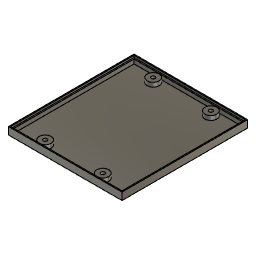
VersaTermBottom (Autodesk Fusion 360 design; units mm, degrees)
Autodesk Fusion 360 part; units mm, degrees
box "BoxPrimitive1" add length 104.5 width 94.5 height 5.5 placed x (0, 1, 0) y (-1, 0, 0) z (0, 0, 1) at (94.5, 0, 0) makes body 1
shell "Shell1" thickness 2 removed faces 1 at (31.5, 34.8333, 5.5) on bodies 1
sketch "Sketch3" plane through (0, 0, 2) normal (0, 0, 1) x (-1, 0, 0)
  line L0 (-92.5, -102.5) -> (-2, -102.5)
  line L1 (-2, -102.5) -> (-2, -2)
  line L2 (-2, -2) -> (-92.5, -2)
  line L3 (-92.5, -2) -> (-92.5, -102.5)
  circle A0 centre (-23.25, -97.25) radius 5
  dimension "d7" = 10
  dimension "d8" = 5.25
  dimension "d9" = 21.25
  measures "d7" diameter of A0
  measures "d8" distance of L0 A0.centre
  measures "d9" distance of L1 A0.centre
extrude "Extrude1" add sketch "Sketch3" along normal blind 3.5 contours A0 bodies 1
sketch "Sketch6" plane through (0, 0, 0) normal (0, 0, -1) x (1, 0, 0)
  line L0 (0, -104.5) -> (94.5, -104.5)
  line L1 (94.5, -104.5) -> (94.5, 0)
  line L2 (94.5, 0) -> (0, 0)
  line L3 (0, 0) -> (0, -104.5)
  line L4 (19.8436, -97.25) -> (21.5468, -100.2)
  line L5 (21.5468, -100.2) -> (24.9532, -100.2)
  line L6 (24.9532, -100.2) -> (26.6564, -97.25)
  line L7 (26.6564, -97.25) -> (24.9532, -94.3)
  line L8 (24.9532, -94.3) -> (21.5468, -94.3)
  line L9 (21.5468, -94.3) -> (19.8436, -97.25)
  point P0 (23.25, -97.25)
  dimension "d12" = 2.95
  dimension "d13" = 23.25
  dimension "d14" = 7.25
  constraint horizontal L5
  measures "d12" distance of P0 L4
  measures "d13" distance of L3 P0
  measures "d14" distance of L0 P0
extrude "Extrude2" cut sketch "Sketch6" against normal blind 3.5 contours L4 L5 L6 L7 L8 L9 bodies 1
sketch "Sketch9" plane through (0, 0, 5.5) normal (0, 0, 1) x (-1, 0, 0)
  circle A0 centre (-23.25, -97.25) radius 5
  circle A1 centre (-23.25, -97.25) radius 1.6
  dimension "d18" = 3.2
  constraint concentric A0 A1
  measures "d18" diameter of A1
extrude "Extrude3" cut sketch "Sketch9" against normal blind 5 contours A1 bodies 1
pattern_linear "R-Pattern1" count 2 spacing 48 along (1, 0, 0) count 2 spacing 90 along (0, -1, 0) of "Extrude1", "Extrude2", "Extrude3"
sketch "Sketch12" plane through (0, 0, 5.5) normal (0, 0, 1) x (-1, 0, 0)
  line L0 (-92.5, -102.5) -> (-92.5, -2)
  line L1 (-92.5, -2) -> (-2, -2)
  line L2 (-2, -2) -> (-2, -102.5)
  line L3 (-2, -102.5) -> (-92.5, -102.5)
  line L4 (-94.5, -104.5) -> (0, -104.5)
  line L5 (0, -104.5) -> (0, 0)
  line L6 (0, 0) -> (-94.5, 0)
  line L7 (-94.5, 0) -> (-94.5, -104.5)
  line L8 (0, -104.5) -> (-94.5, -104.5)
  line L9 (-94.5, -104.5) -> (-94.5, 0)
  line L10 (-94.5, 0) -> (0, 0)
  line L11 (0, 0) -> (0, -104.5)
  line L12 (-0.9, -0.9) -> (-0.9, -103.6)
  line L13 (-0.9, -103.6) -> (-93.6, -103.6)
  line L14 (-93.6, -103.6) -> (-93.6, -0.9)
  line L15 (-93.6, -0.9) -> (-0.9, -0.9)
  dimension "d26" = 0.9
  constraint horizontal L8
  constraint vertical L9
  constraint horizontal L10
  constraint vertical L11
  constraint coincident L6.end L7.start
  constraint coincident L4.end L5.start
extrude "Extrude4" add sketch "Sketch12" along normal blind 1.6 separate body contours L4 L5 L6 L7 L8 L9 L10 L11 makes body 2
chamfer "Chamfer1" distance 1 angle 45 4 edges at (47.25, 104.5, 0) (0, 52.25, 0) (94.5, 52.25, 0) (47.25, 0, 0) on bodies 1
combine "Combine1" operation add target body 1 tool bodies 2
